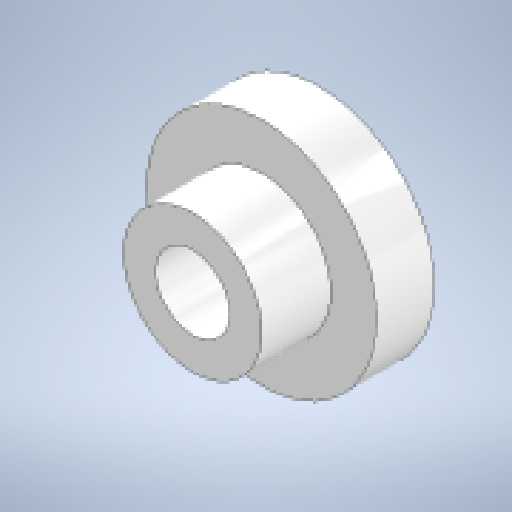
# Autodesk Inventor part: suberase
Saved by Autodesk Inventor 2025.1 (Build 291241000, 241)
## iProperties
Created: 2024-09-01
Part Number: suberase
Material: ABS プラスチック
Document SubType Name: Modeling
Designer: right
Density: 1.06 g/cm^3
Appearance: 滑らか - 白
Mass: 0.251155 g
Surface Area: 3.31375 cm^2
Volume: 0.236939 cm^3
Author: right
Autodesk Inventor part; units mm, degrees
ref_plane "YZ Plane" through (0, 0, 0) normal (1, 0, 0) x (0, 1, 0)
sketch "スケッチ1" plane through (0, 0, 0) normal (0, 0, 1) x (1, 0, 0)
  circle A0 centre (4.9656, 36.5874) radius 1.3 projected
  circle A1 centre (4.9656, 36.5874) radius 5
  circle A2 centre (4.9656, 36.5874) radius 3
  circle A3 centre (4.9656, 36.5874) radius 1.6
  point P0 (0, 0)
  dimension "d0" = 10
  dimension "d1" = 6
  dimension "d2" = 3.2
  constraints: 3 centre point, 3 coincident
  measures "d0" diameter of A1
  measures "d1" diameter of A2
  measures "d2" diameter of A3
ref_plane "作業平面1" through (-16.355, -22.2242, 2.5) normal (0, 0, -1) x (-0.6765, 0.7365, 0)
extrude "押し出し1" add sketch "スケッチ1" along normal up to surface (2.5 mm away) contours A1 | A2
sketch "スケッチ2" plane through (4.9656, 36.5874, 2.5) normal (0, 0, 1) x (1, 0, 0)
  circle A0 centre (0, 0) radius 1.6 projected
  circle A1 centre (0, 0) radius 1.6
  circle A2 centre (0, 0) radius 3
  point P0 (-4.9656, -36.5874)
  dimension "d5" = 3.2
  dimension "d6" = 6
  constraints: 2 centre point, 2 coincident
  measures "d5" diameter of A1
  measures "d6" diameter of A2
ref_plane "作業平面2" through (-16.355, -22.2242, 5.5) normal (0, 0, 1) x (0.7365, 0.6765, 0)
extrude "押し出し2" add sketch "スケッチ2" along normal up to surface (3 mm away)
